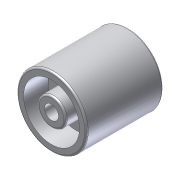
# Autodesk Inventor part: Conveyor_Roller_MainOuter
Saved by Autodesk Inventor 2012 (Build 160160000, 160)
## iProperties
Created: 2012-01-14
Part Number: Conveyor_Roller_MainOuter
Material: PVC-Piping
Document SubType Name: Modeling
Designer: JesseK
Density: 1.4 g/cm^3
Mass: 25.2865 g
Surface Area: 82.644 cm^2
Volume: 18.0618 cm^3
Author: JesseK
Autodesk Inventor part; units mm, degrees
ref_plane "YZ Plane" through (0, 0, 0) normal (1, 0, 0) x (0, 1, 0)
ref_plane "XZ Plane" through (0, 0, 0) normal (0, 1, 0) x (-1, 0, 0)
ref_plane "XY Plane" through (0, 0, 0) normal (0, 0, 1) x (1, 0, 0)
sketch "Sketch1" plane through (0, 0, 0) normal (0, 0, 1) x (1, 0, 0)
  circle A0 centre (0, 0) radius 15.875
  circle A1 centre (0, 0) radius 3.175
  dimension "d0" = 31.75
  dimension "d1" = 6.35
  constraints: 2 centre point, 2 coincident
  measures "d0" diameter of A0
  measures "d1" diameter of A1
extrude "Extrusion1" add sketch "Sketch1" along normal blind 34.925
sketch "Sketch2" plane through (0, 0, 34.925) normal (0, 0, 1) x (1, 0, 0)
  circle A0 centre (0, 0) radius 15.875 projected
  circle A1 centre (0, 0) radius 6.35
  circle A2 centre (0, 0) radius 12.7
  dimension "d4" = 6.35
  dimension "d5" = 12.7
  constraints: 2 centre point, 2 coincident
  measures "d4" radial gap between concentric circles of A2 A1
  measures "d5" diameter of A1
extrude "Extrusion2" cut sketch "Sketch2" against normal blind 11.1125 contours A2
sketch "Sketch3" plane through (0, 0, 0) normal (0, 0, -1) x (-1, 0, 0)
  circle A0 centre (0, 0) radius 15.875 projected
  circle A1 centre (0, 0) radius 6.35
  circle A2 centre (0, 0) radius 12.7
  dimension "d8" = 12.7
  dimension "d9" = 6.35
  constraints: 2 centre point, 2 coincident
  measures "d8" diameter of A1
  measures "d9" radial gap between concentric circles of A1 A2
extrude "Extrusion3" cut sketch "Sketch3" against normal blind 11.1125 contours A2
fillet "Fillet1" radius 0.7937 4 edges at (6.35, 0, 0) (-15.875, 0, 0) (-6.35, 0, 34.925) (-15.875, 0, 34.925)
body "Solid1"
